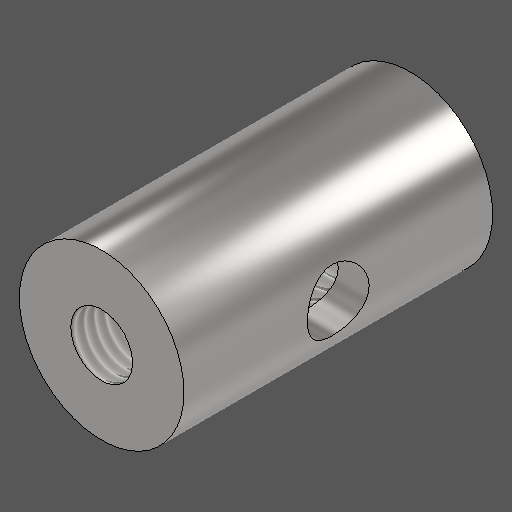
# Autodesk Inventor part: anode-bushing-adapter
Saved by Autodesk Inventor 2025 (Build 290162000, 162)
## iProperties
Created: 2024-05-16
Part Number: anode-bushing-adapter
Material: Stainless Steel
Document SubType Name: Modeling
Designer: kuzmin
Density: 8 g/cm^3
Appearance: Semi-Polished
Author: kuzmin
Autodesk Inventor part; units mm, degrees
ref_plane "YZ Plane" through (0, 0, 0) normal (1, 0, 0) x (0, 1, 0)
ref_plane "XZ Plane" through (0, 0, 0) normal (0, 1, 0) x (-1, 0, 0)
ref_plane "XY Plane" through (0, 0, 0) normal (0, 0, 1) x (1, 0, 0)
sketch "Sketch1" plane through (0, 0, 0) normal (0, 1, 0) x (-1, 0, 0)
  line L0 (4, 7.5) -> (1.5, 7.5)
  line L1 (2.5, -7.5) -> (4, -7.5)
  line L2 (4, -7.5) -> (4, 7.5)
  line L3 (1.5, 7.5) -> (0, 7.5) construction
  line L4 (0, 7.5) -> (0, -7.5)
  line L5 (0, -7.5) -> (2.5, -7.5) construction
  line L6 (2.5, -7.5) -> (2.5, 2.5)
  line L7 (2.5, 2.5) -> (1.5, 2.5)
  line L8 (1.5, 2.5) -> (1.5, 7.5)
  point P0 (0, 0)
  point P1 (0, 0)
  dimension "d0" = 8
  dimension "d2" = 15
  dimension "d4" = 5
  dimension "d5" = 3
  dimension "d6" = 5
  constraints: 18 end point, 4 perpendicular, 2 horizontal, 1 coincident, 1 midpoint, 1 parallel, 1 vertical
  measures "d0" diameter of L2 L4
  measures "d2" distance of L1.end L0.start
  measures "d4" diameter of L6 L4
  measures "d5" diameter of L8 L4
  measures "d6" distance of L7.end L0.end
revolve "Revolution1" add sketch "Sketch1" angle 360 about axis through (0, 0, 7.5) along (0, 0, -1)
thread "Thread1" size "M5x0.8" class "6H" standard "ANSI Metric M Profile" full length
thread "Thread2" size "M3x0.5" class "6H" standard "ANSI Metric M Profile" full length
sketch "Sketch2" plane through (0, 0, 0) normal (1, 0, 0) x (0, 1, 0)
  circle A0 centre (0, 0) radius 1.5
  dimension "d11" = 3
  constraints: 1 centre point, 1 coincident
  measures "d11" diameter of A0
extrude "Extrusion1" cut sketch "Sketch2" along normal through all both and the other way through all
body "Solid1"
